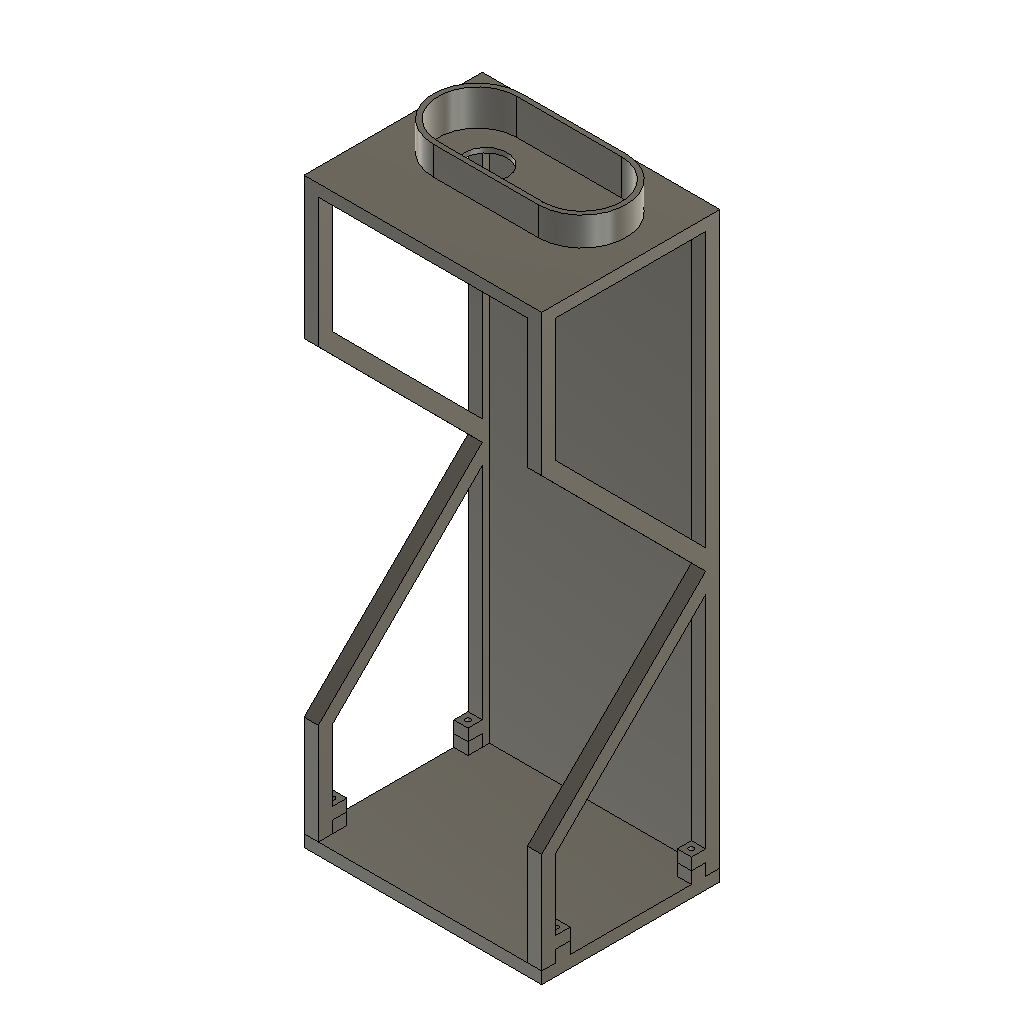
color-detector (Autodesk Fusion 360 design; units mm, degrees)
Autodesk Fusion 360 part; units mm, degrees
note: some values were not read from the file. Chosen so that the rebuilt part matches the saved one: which bodies a step acts on.
sketch "Sketch1" plane through (0, 0, 0) normal (0, 0, 1) x (1, 0, 0)
  line L0 (50, 37.5) -> (-50, 37.5)
  line L1 (-50, 37.5) -> (-50, -37.5)
  line L2 (-50, -37.5) -> (50, -37.5)
  line L3 (50, -37.5) -> (50, 37.5)
  line L4 (50, 37.5) -> (-50, -37.5) construction
  line L5 (-50, 37.5) -> (50, -37.5) construction
  dimension "d1" = 100
  dimension "d2" = 75
  constraint horizontal L0
  constraint perpendicular L0 L1
  constraint parallel L0 L2
  constraint parallel L1 L3
  constraint coincident L4 origin
  constraint coincident L5 origin
  measures "d1" distance of L1.end L2.end
  measures "d2" distance of L0.end L1.end
extrude "Extrude1" add sketch "Sketch1" along normal blind 5 makes body 1
sketch "Sketch2" plane through (0, 0, 5) normal (0, 0, 1) x (-1, 0, 0)
  line L0 (-50, 37.5) -> (-50, -37.5)
  line L1 (-50, -37.5) -> (50, -37.5)
  line L2 (50, -37.5) -> (50, 37.5)
  line L3 (50, 37.5) -> (-50, 37.5)
  line L4 (42, -31.5) -> (50, -31.5)
  line L5 (50, 37.5) -> (44, 37.5)
  line L6 (44, 37.5) -> (44, 31.5)
  line L7 (44, 31.5) -> (50, 31.5)
  line L8 (50, 31.5) -> (50, 37.5)
  line L9 (-50, 37.5) -> (-44, 37.5)
  line L10 (-44, 37.5) -> (-44, 31.5)
  line L11 (-44, 31.5) -> (-50, 31.5)
  line L12 (-50, 31.5) -> (-50, 37.5)
  line L13 (-42, -31.5) -> (-50, -31.5)
  line L14 (-50, -31.5) -> (-44, -31.5)
  line L15 (-44, -31.5) -> (-44, -25.5)
  line L16 (-44, -25.5) -> (-50, -25.5)
  line L17 (-50, -25.5) -> (-50, -31.5)
  line L18 (-50, 31.5) -> (-44, 31.5)
  line L19 (-44, 31.5) -> (-44, 25.5)
  line L20 (-44, 25.5) -> (-50, 25.5)
  line L21 (-50, 25.5) -> (-50, 31.5)
  line L22 (50, 31.5) -> (44, 31.5)
  line L23 (44, 31.5) -> (44, 25.5)
  line L24 (44, 25.5) -> (50, 25.5)
  line L25 (50, 25.5) -> (50, 31.5)
  line L26 (50, -31.5) -> (44, -31.5)
  line L27 (44, -31.5) -> (44, -25.5)
  line L28 (44, -25.5) -> (50, -25.5)
  line L29 (50, -25.5) -> (50, -31.5)
  line L30 (-50, -31.5) -> (50, -31.5)
  line L31 (50, -31.5) -> (50, -37.5)
  line L32 (50, -37.5) -> (-50, -37.5)
  line L33 (-50, -37.5) -> (-50, -31.5)
  line L34 (-42, -31.5) -> (42, -31.5)
  line L35 (42, -31.5) -> (42, -34.5)
  line L36 (42, -34.5) -> (-42, -34.5)
  line L37 (-42, -34.5) -> (-42, -31.5)
  dimension "d6" = 6
  dimension "d7" = 6
  dimension "d8" = 6
  dimension "d9" = 6
  dimension "d10" = 6
  dimension "d12" = 6
  dimension "d13" = 6
  dimension "d14" = 6
  dimension "d15" = 6
  dimension "d16" = 6
  dimension "d17" = 6
  dimension "d18" = 6
  dimension "d19" = 6
  dimension "d20" = 6
  dimension "d21" = 84
  dimension "d22" = 3
  constraint horizontal L4
  constraint horizontal L5
  constraint vertical L6
  constraint horizontal L7
  constraint vertical L8
  constraint coincident L2.end L3.start
  constraint horizontal L9
  constraint vertical L10
  constraint horizontal L11
  constraint vertical L12
  constraint coincident L0.start L3.end
  constraint horizontal L13
  constraint horizontal L14
  constraint vertical L15
  constraint horizontal L16
  constraint vertical L17
  constraint horizontal L18
  constraint vertical L19
  constraint horizontal L20
  constraint vertical L21
  constraint horizontal L22
  constraint vertical L23
  constraint horizontal L24
  constraint vertical L25
  constraint horizontal L26
  constraint vertical L27
  constraint horizontal L28
  constraint vertical L29
  constraint horizontal L30
  constraint vertical L31
  constraint horizontal L32
  constraint vertical L33
  constraint coincident L1.end L2.start
  constraint horizontal L34
  constraint vertical L35
  constraint horizontal L36
  constraint vertical L37
  measures "d6" distance of L1.end L4.end
  measures "d7" distance of L2.end L5.end
  measures "d8" distance of L2.end L7.end
  measures "d9" distance of L0.start L9.end
  measures "d10" distance of L0.start L11.end
  measures "d12" distance of L0.end L13.end
  measures "d13" distance of L13.end L14.end
  measures "d14" distance of L13.end L16.end
  measures "d15" distance of L11.end L10.end
  measures "d16" distance of L11.end L20.end
  measures "d17" distance of L7.end L6.end
  measures "d18" distance of L7.end L24.end
  measures "d19" distance of L4.end L26.end
  measures "d20" distance of L4.end L28.end
  measures "d21" distance of L13.start L4.start
  measures "d22" distance of L13.start L36.end
extrude "Extrude2" add sketch "Sketch2" along normal blind 300 separate body contours L0 L3 L9 L10 L11 L12 L18 | L2 L3 L5 L6 L7 L8 L22 | L0 L1 L2 L4 L13 L14 L26 L30 L31 L32 L33 L35 L36 L37 makes body 2 at (46, -37.5, 105) makes body 3 at (16.6667, 37.5, 105) makes body 4 at (-48, -37.5, 105)
sketch "Sketch3" plane through (0, 0, 305) normal (0, 0, 1) x (-1, 0, 0)
  line L0 (42, -31.5) -> (42, -34.5)
  line L1 (42, -34.5) -> (-42, -34.5)
  line L2 (-42, -34.5) -> (-42, -31.5)
  line L3 (-42, -31.5) -> (-50, -31.5)
  line L4 (-50, -31.5) -> (-50, -37.5)
  line L5 (-50, -37.5) -> (50, -37.5)
  line L6 (50, -37.5) -> (50, -31.5)
  line L7 (50, -31.5) -> (42, -31.5)
  line L8 (50, -37.5) -> (-50, -37.5)
  line L9 (-50, -37.5) -> (-50, 37.5)
  line L10 (-50, 37.5) -> (50, 37.5)
  line L11 (50, 37.5) -> (50, -37.5)
  dimension "d25" = 100
  dimension "d26" = 75
  constraint horizontal L8
  constraint vertical L9
  constraint horizontal L10
  constraint vertical L11
  constraint coincident L5.end L6.start
  measures "d1" distance of L5.end L4.end
extrude "Extrude3" add sketch "Sketch3" along normal blind 5 bodies 2 3 4
sketch "Sketch4" plane through (0, 0, 310) normal (0, 0, 1) x (-1, 0, 0)
  line L0 (50, 37.5) -> (-50, 37.5)
  line L1 (-50, 37.5) -> (-50, -37.5)
  line L2 (-50, -37.5) -> (50, -37.5)
  line L3 (50, -37.5) -> (50, 37.5)
  line L4 (-37, -7.5) -> (37, -7.5)
  line L5 (22, 9) -> (-22, 9)
  arc A0 (-22, 9) -> (-22, -24) centre (-22, -7.5) ccw
  line L6 (-22, -24) -> (22, -24)
  arc A1 (22, -24) -> (22, 9) centre (22, -7.5) ccw
  line L7 (22, -7.5) -> (-22, -7.5) construction
  line L8 (22, 11) -> (-22, 11)
  arc A2 (-22, 11) -> (-22, -26) centre (-22, -7.5) ccw
  line L9 (-22, -26) -> (22, -26)
  arc A3 (22, -26) -> (22, 11) centre (22, -7.5) ccw
  point P0 (-22, -7.5)
  point P1 (0, -7.5)
  point P2 (0, -7.5)
  dimension "d29" = 74
  dimension "d30" = 13
  dimension "d31" = 30
  dimension "d32" = 22
  dimension "d33" = 33
  dimension "d34" = 2
  constraint horizontal L4
  constraint coincident L4 P0
  constraint midpoint L4 P2
  constraint tangent L5 A0
  constraint tangent A0 L6
  constraint parallel L5 L6
  constraint tangent L6 A1
  constraint tangent L5 A1
  constraint coincident P0 A0.centre
  constraint parallel L4 L7
  constraint coincident P2 P1
  constraint midpoint L7 P2
  measures "d29" distance of L4.start L4.end
  measures "d30" distance of L1 L4.start
  measures "d31" distance of L2 L4
  measures "d32" distance of P0 P2
  measures "d33" diameter of A0
extrude "Extrude4" cut sketch "Sketch4" against normal blind 3 contours L5 A0 L6 A1 bodies 2
extrude "Extrude5" add sketch "Sketch4" along normal blind 12 contours L8 A2 L9 A3 bodies 2
sketch "Sketch5" plane through (0, 0, 307) normal (0, 0, 1) x (-1, 0, 0)
  arc A0 (22, -24) -> (22, 9) centre (22, -7.5) ccw
  line L0 (22, 9) -> (-22, 9)
  arc A1 (-22, 9) -> (-22, -24) centre (-22, -7.5) ccw
  line L1 (-22, -24) -> (22, -24)
  circle A2 centre (18.5, -7.5) radius 9
  point P0 (0, -7.5)
  dimension "d39" = 18
  dimension "d40" = 16.5
  dimension "d41" = 16.5
  dimension "d42" = 18.5
  measures "d39" diameter of A2
  measures "d40" distance of L0 P0
  measures "d41" distance of L0 A2.centre
  measures "d42" distance of A2.centre P0
extrude "Extrude6" cut sketch "Sketch5" against normal blind 15 contours A2 bodies 2
extrude "Extrude7" add sketch "Sketch2" along normal blind 5 separate body contours L0 L11 L18 L19 L20 L21 | L0 L13 L14 L15 L16 L17 L30 | L2 L7 L22 L23 L24 L25 | L2 L4 L26 L27 L28 L29 L30 makes body 5 at (-46, 29.5, 5) makes body 6 at (-46, -27.5, 5) makes body 7 at (48, 29.5, 5) makes body 8 at (48, -27.5, 5)
combine "Combine1" operation add target body 1 tool bodies 5 6 7 8
extrude "Extrude8" add 4 faces at (-46, 29.5, 10) (-46, -27.5, 10) (48, 29.5, 10) (48, -27.5, 10) along direction (0, 0, 1) blind 5 separate body on bodies 1 makes body 9 at (48, 29.5, 10) makes body 10 at (-46, 29.5, 10) makes body 11 at (-46, -27.5, 10) makes body 12 at (48, -27.5, 10)
combine "Combine2" operation add target body 2 tool bodies 9 10 11 12
extrude "Extrude9" cut 1 faces at (-42, 32.5, 205) along direction (-1, 0, 0) blind 2 on bodies 2 bodies 2
extrude "Extrude10" cut 1 faces at (42, 33.5, 205) along direction (1, 0, 0) blind 2 on bodies 2 bodies 2
sketch "Sketch6" plane through (0, 0, 15) normal (0, 0, 1) x (-1, 0, 0)
  line L0 (-50, -31.5) -> (-44, -31.5)
  line L1 (-44, -31.5) -> (-44, -25.5)
  line L2 (-44, -25.5) -> (-50, -25.5)
  line L3 (-50, -25.5) -> (-50, -31.5)
  line L4 (-44, -25.5) -> (44, -25.5)
  line L5 (44, -25.5) -> (44, 25.5)
  line L6 (44, 25.5) -> (-44, 25.5)
  line L7 (-44, 25.5) -> (-44, -25.5)
  dimension "d53" = 88
  dimension "d54" = 51
  constraint horizontal L4
  constraint vertical L5
  constraint horizontal L6
  constraint vertical L7
  constraint coincident L1.end L2.start
  measures "d53" distance of L1.end L4.end
  measures "d54" distance of L1.end L6.end
sketch "Sketch7" plane through (0, 0, 15) normal (0, 0, 1) x (-1, 0, 0)
  line L0 (-50, -31.5) -> (-44, -31.5)
  line L1 (-44, -31.5) -> (-44, -25.5)
  line L2 (-44, -25.5) -> (-50, -25.5)
  line L3 (-50, -25.5) -> (-50, -31.5)
  circle A0 centre (-47, -28.5) radius 1.05
  line L4 (-50, -25.5) -> (-50, -31.5)
  circle A1 centre (47, -28.5) radius 1.05
  circle A2 centre (-47, 28.5) radius 1.05
  circle A3 centre (47, 28.5) radius 1.05
  dimension "d55" = 2.1
  dimension "d56" = 3
  dimension "d57" = 3
  dimension "d60" = 94
  dimension "d61" = 57
  measures "d55" diameter of A0
  measures "d56" distance of L2 A0.centre
  measures "d57" distance of A0.centre L4
extrude "Extrude11" cut sketch "Sketch7" against normal blind 10 contours A0 | A1 | A2 | A3 bodies 1 2
sketch "Sketch8" plane through (0, 0, 310) normal (0, 0, 1) x (-1, 0, 0)
  line L0 (22, -26) -> (-22, -26)
  arc A0 (-22, 11) -> (-22, -26) centre (-22, -7.5) ccw
  line L1 (-22, 11) -> (22, 11)
  arc A1 (22, -26) -> (22, 11) centre (22, -7.5) ccw
  line L2 (50, 37.5) -> (-50, 37.5)
  line L3 (-50, 37.5) -> (-50, -37.5)
  line L4 (-50, -37.5) -> (50, -37.5)
  line L5 (50, -37.5) -> (50, 37.5)
  line L6 (61.4973, -41.8459) -> (-74.4441, -41.8459)
  line L7 (-74.4441, -41.8459) -> (-74.4441, 59.4166)
  line L8 (-74.4441, 59.4166) -> (61.4973, 59.4166)
  line L9 (61.4973, 59.4166) -> (61.4973, -41.8459)
  constraint horizontal L6
  constraint vertical L7
  constraint horizontal L8
  constraint vertical L9
extrude "Extrude12" cut sketch "Sketch8" along normal blind -150 and the other way blind 85 contours L2 L3 L4 L5 bodies 2 makes body 13 at (16.6667, 37.5, 253.3333) makes body 14 at (44, -35.5, 60) makes body 15 at (16.6667, 37.5, 56.6667)
move_body "Move1" bodies 13 to x (1, 0, 0) y (0, 1, 0) z (0, 0, 1) at (0, 0, -65)
combine "Combine3" operation add target body 2 tool bodies 14 15 13
sketch "Sketch9" plane through (50, 0, 0) normal (1, 0, 0) x (0, 1, 0)
  line L0 (-37.5, 245) -> (-37.5, 5)
  line L1 (-37.5, 5) -> (-31.5, 5)
  line L2 (-31.5, 5) -> (-31.5, 10)
  line L3 (-31.5, 10) -> (-25.5, 10)
  line L4 (-25.5, 10) -> (-25.5, 15)
  line L5 (-25.5, 15) -> (-31.5, 15)
  line L6 (-31.5, 15) -> (-31.5, 240)
  line L7 (-31.5, 240) -> (31.5, 240)
  line L8 (31.5, 240) -> (31.5, 15)
  line L9 (31.5, 15) -> (25.5, 15)
  line L10 (25.5, 15) -> (25.5, 10)
  line L11 (25.5, 10) -> (31.5, 10)
  line L12 (31.5, 10) -> (31.5, 5)
  line L13 (31.5, 5) -> (37.5, 5)
  line L14 (37.5, 5) -> (37.5, 245)
  line L15 (37.5, 245) -> (-37.5, 245)
  line L16 (-31.5, 5) -> (-31.5, 45)
  line L17 (-31.5, 45) -> (-35.7325, 49.2528)
  line L18 (-35.7325, 49.2528) -> (33.4827, 118.1381)
  line L19 (33.4827, 118.1381) -> (37.5, 114.1015)
  line L20 (37.5, 113.6712) -> (-31.5, 45)
  line L21 (-35.7325, 49.2528) -> (-37.5, 47.4937)
  line L22 (31.5, 116.1649) -> (35.7528, 120.3974)
  line L23 (35.7528, 120.3974) -> (-33.7297, 190.2125)
  line L24 (-33.7297, 190.2125) -> (-37.5, 186.4602)
  line L25 (-37.5, 185.4953) -> (31.5, 116.1649)
  dimension "d69" = 40
  dimension "d70" = 6
  dimension "d71" = 6
  constraint vertical L16
  constraint coincident L1.end L2.start
  constraint perpendicular L17 L18
  constraint parallel L17 L19
  constraint parallel L18 L20
  constraint perpendicular L17 L21
  constraint coincident L0 L21.end
  constraint perpendicular L22 L23
  constraint parallel L22 L24
  constraint parallel L23 L25
  constraint perpendicular L19 L22
  constraint coincident L8 L22.start
  constraint coincident L18 L22.start
  constraint coincident L0 L24.end
  constraint coincident L0 L25.start
  constraint coincident L14 L19.end
  constraint coincident L14 L20.start
  measures "d69" distance of L1.end L16.end
  measures "d70" distance of L17.end L16.end
  measures "d71" distance of L22.start L22.end
extrude "Extrude13" cut sketch "Sketch9" against normal blind 110 contours L0 L6 L18 L21 L25 bodies 2 makes body 16 at (-16.6667, 37.5, 165) makes body 17 at (-44, -35.5, 22.4979)
extrude "Extrude14" add sketch "Sketch9" against normal blind 6 contours L6 L8 L23 L25 | L6 L8 L18 L20 bodies 2 16
extrude "Extrude15" add sketch "Sketch9" along normal blind -94 and the other way blind 100 contours L6 L8 L23 L25 | L6 L8 L18 L20 bodies 2 17
named bodies: "base", "top", "TopWithLegs (1)", "TopWithLegs (2)", "TopWithLegs (3)", "top (1)", "top (2)"
